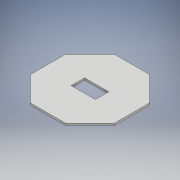
# Autodesk Inventor part: TopR01
Saved by Autodesk Inventor 2018.1 (Build 221171000, 171)
## iProperties
Created: 2017-10-23
Part Number: TopR01
Material: Generic
Document SubType Name: Modeling
Designer: s167968
Density: 1 g/cm^3
Appearance: Default
Author: s167968
Autodesk Inventor part; units mm, degrees
ref_plane "YZ Plane" through (0, 0, 0) normal (1, 0, 0) x (0, 1, 0)
ref_plane "XZ Plane" through (0, 0, 0) normal (0, 1, 0) x (-1, 0, 0)
ref_plane "XY Plane" through (0, 0, 0) normal (0, 0, 1) x (1, 0, 0)
sketch "Sketch1" plane through (0, 0, 0) normal (0, 0, 1) x (1, 0, 0)
  line L0 (37.4203, -15.5) -> (15.5, -37.4203)
  line L1 (15.5, -37.4203) -> (-15.5, -37.4203)
  line L2 (-15.5, -37.4203) -> (-37.4203, -15.5)
  line L3 (-37.4203, -15.5) -> (-37.4203, 15.5)
  line L4 (-37.4203, 15.5) -> (-15.5, 37.4203)
  line L5 (-15.5, 37.4203) -> (15.5, 37.4203)
  line L6 (15.5, 37.4203) -> (37.4203, 15.5)
  line L7 (37.4203, 15.5) -> (37.4203, -15.5)
  point P0 (0, 0)
  point P1 (0, 0)
  point P2 (0, 0)
  dimension "d0" = 31
  dimension "d1" = 0
  constraints: 16 end point, 1 coincident, 17 other
  measures "d0" distance of L4.end L5.end
  measures "d1" vertical distance of L4.end L5.end
extrude "Extrusion1" add sketch "Sketch1" along normal blind 2
sketch "Sketch2" plane through (0, 0, 2) normal (0, 0, 1) x (1, 0, 0)
  line L0 (-10.75, 6) -> (10.75, 6)
  line L1 (10.75, 6) -> (10.75, -6)
  line L2 (10.75, -6) -> (-10.75, -6)
  line L3 (-10.75, -6) -> (-10.75, 6)
  point P0 (0, 0)
  dimension "d5" = 21.5
  dimension "d6" = 12
  dimension "d7" = 10.75
  dimension "d8" = 6
  constraints: 8 end point, 2 parallel, 1 horizontal, 1 perpendicular
  measures "d5" distance of L0.start L0.end
  measures "d6" distance of L2.end L0.start
  measures "d7" distance from line of L3 point (0, 0)
  measures "d8" distance from line of L0 point (0, 0)
extrude "Extrusion2" cut sketch "Sketch2" against normal blind 3
equation "\"d7\" = 0.5 * d5"
equation "\"d8\" = 0.5 * d6"
body "Solid1"
